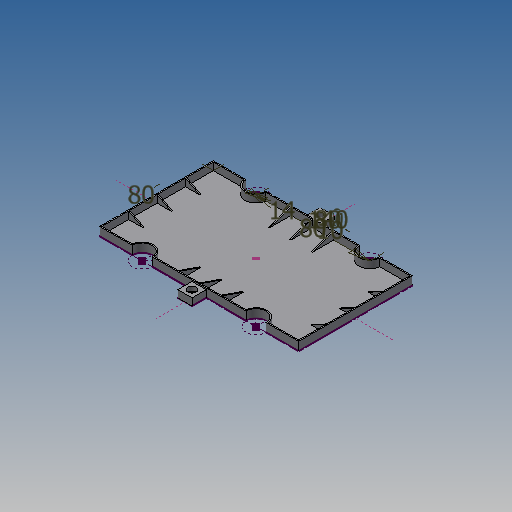
# Autodesk Inventor part: Leste_Meca_IIm_Ligne
Saved by Autodesk Inventor 2025.3 (Build 293356000, 356)
## iProperties
Created: 2026-08-27
Part Number: Leste_Meca_IIm_Ligne
Project: Nom Projet
Material: .
Description: Nom pièce
Document SubType Name: Modeling
Designer: jules
Authority: brut Ø
Mass: 0.0117645 g
Surface Area: 284.842 cm^2
Volume: 11.7645 cm^3
Density: 0.001 g/cm^3
Appearance: Par défaut
Material number: ---
Author: jules
Autodesk Inventor part; units mm, degrees
ref_plane "Plan YZ" through (0, 0, 0) normal (1, 0, 0) x (0, 1, 0)
ref_plane "Plan XZ" through (0, 0, 0) normal (0, 1, 0) x (-1, 0, 0)
ref_plane "Plan XY" through (0, 0, 0) normal (0, 0, 1) x (1, 0, 0)
sketch "Esquisse1" plane through (0, 0, 0) normal (0, 0, 1) x (1, 0, 0)
  line L0 (70, -40) -> (-70, -40) construction
  line L1 (-70, -40) -> (-70, 40)
  line L2 (-70, 40) -> (70, 40) construction
  line L3 (70, 40) -> (70, -40)
  line L4 (70, -40) -> (-70, 40) construction
  line L5 (-70, -40) -> (70, 40) construction
  line L6 (40, -40) -> (-40, -40) construction
  line L7 (-40, -40) -> (-40, 40) construction
  line L8 (-40, 40) -> (40, 40) construction
  line L9 (40, 40) -> (40, -40) construction
  line L10 (40, -40) -> (-40, 40) construction
  line L11 (-40, -40) -> (40, 40) construction
  circle A0 centre (-40, 40) radius 7 construction
  line L12 (-98, 0) -> (98, 0) construction
  arc A1 (-47, 40) -> (-33, 40) centre (-40, 40) ccw
  circle A2 centre (40, 40) radius 7 construction
  arc A3 (33, 40) -> (47, 40) centre (40, 40) ccw
  circle A4 centre (-40, -40) radius 7 construction
  arc A5 (-33, -40) -> (-47, -40) centre (-40, -40) ccw
  circle A6 centre (40, -40) radius 7 construction
  arc A7 (47, -40) -> (33, -40) centre (40, -40) ccw
  line L13 (-47, 40) -> (-70, 40)
  line L14 (-33, 40) -> (33, 40)
  line L15 (47, 40) -> (70, 40)
  line L16 (-70, -40) -> (70, -40) construction
  line L17 (-47, -40) -> (-70, -40)
  line L18 (-33, -40) -> (33, -40)
  line L19 (47, -40) -> (70, -40)
  line L20 (0, -70) -> (0, 70) construction
  line L21 (-5, 40) -> (5, 40)
  line L22 (5, 40) -> (5, 50)
  line L23 (5, 50) -> (-5, 50)
  line L24 (-5, 50) -> (-5, 40)
  line L25 (-5, 40) -> (5, 50) construction
  line L26 (5, 40) -> (-5, 50) construction
  line L27 (-70, -40) -> (70, -40) construction
  line L28 (-40, -40) -> (40, -40) construction
  line L29 (-33, -40) -> (33, -40)
  line L30 (5, -40) -> (5, -50)
  line L31 (5, -50) -> (-5, -50)
  line L32 (-5, -50) -> (-5, -40)
  point P0 (0, 0)
  point P1 (0, 45)
  dimension "d0" = 140
  dimension "d1" = 80
  dimension "d2" = 80
  dimension "d3" = 14
  dimension "d13" = 80
  dimension "d34" = 10
  dimension "d35" = 10
  constraints: 62 end point, 17 point on circle, 14 symmetric about line, 8 centre point, 6 midpoint, 6 parallel, 6 point on line, 4 collinear, 4 horizontal, 3 perpendicular, 1 coincident, 1 concentric, 1 vertical, 10 other
  measures "d0" distance of L1.end L2.end
  measures "d1" distance of L0.end L1.end
  measures "d2" distance of L7.end L8.end
  measures "d3" diameter of A0
  measures "d13" distance of A0.centre A2.centre
  measures "d34" distance of L23.end L22.end
  measures "d35" distance of L22.end L21.end
extrude "Extrusion1" add sketch "Esquisse1" along normal blind 6 contours L1 L13 A1 L14 A3 L15 L3 L19 A7 L18 A5 L17
shell "Coque1" thickness 0.8 removed faces 1 at (-11.5868, 11.786, 6)
sketch "Esquisse6" plane through (0, 0, 0) normal (1, 0, 0) x (0, 1, 0)
  line L0 (-39.2, 0.8) -> (-32.2, 0.8) construction
  line L1 (-39.2, 0.8) -> (-39.2, 6) construction
  line L2 (39.2, 0.8) -> (-39.2, 0.8) construction
  line L3 (-39.2, 0.8) -> (-39.2, 6) construction
  line L4 (-39.2, 6) -> (-24.2, 0.8)
  line L5 (-39.2, 0.8) -> (-39.2, 6)
  line L6 (-39.2, 0.8) -> (-24.2, 0.8)
  line L7 (0, -1.2) -> (0, 7.2) construction
  line L8 (39.2, 0.8) -> (32.2, 0.8) construction
  line L9 (39.2, 0.8) -> (39.2, 6) construction
  line L10 (-39.2, 0.8) -> (39.2, 0.8) construction
  line L11 (39.2, 0.8) -> (39.2, 6) construction
  line L12 (39.2, 6) -> (24.2, 0.8)
  line L13 (39.2, 0.8) -> (39.2, 6)
  line L14 (39.2, 0.8) -> (24.2, 0.8)
  point P0 (0, 0)
  dimension "d22" = 15
  constraints: 20 end point, 5 symmetric about line, 2 collinear, 2 point on line
  measures "d22" distance of L0.start L4.end
extrude "Extrusion2" add sketch "Esquisse6" along normal mid plane 0.8
pattern_linear "Réseau rectangulaire1" count 3 spacing 15 along (-1, 0, 0) of "Extrusion2" first direction both ways yes
sketch "Esquisse7" plane through (0, 0, 0) normal (0, 1, 0) x (-1, 0, 0)
  line L0 (69.2, 0.8) -> (69.2, 6) construction
  line L1 (47.7589, 0.8) -> (69.2, 0.8) construction
  line L2 (69.2, 6) -> (59.2, 0.8)
  line L3 (69.2, 0.8) -> (69.2, 6)
  line L4 (69.2, 0.8) -> (59.2, 0.8)
  line L5 (0, -1.2) -> (0, 7.2) construction
  line L6 (-69.2, 0.8) -> (-69.2, 6) construction
  line L7 (-47.7589, 0.8) -> (-69.2, 0.8) construction
  line L8 (-69.2, 6) -> (-59.2, 0.8)
  line L9 (-69.2, 0.8) -> (-69.2, 6)
  line L10 (-69.2, 0.8) -> (-59.2, 0.8)
  point P0 (0, 0)
  dimension "d28" = 10
  constraints: 16 end point, 4 symmetric about line, 2 point on line, 1 perpendicular, 1 vertical
  measures "d28" distance from line of L0 L2.end
extrude "Extrusion3" add sketch "Esquisse7" along normal mid plane 0.8
pattern_linear "Réseau rectangulaire2" count 3 spacing 20 along (0, -1, 0) of "Extrusion3" first direction both ways yes
extrude "Extrusion4" add sketch "Esquisse1" along normal blind 5 contours L18 L30 L31 L32 | L24 L23 L22 L14
sketch "Esquisse8" plane through (0, 0, 5) normal (0, 0, 1) x (1, 0, 0)
  line L0 (-5, 40) -> (5, 50) construction
  line L1 (5, 40) -> (-5, 50) construction
  point P0 (0, 0)
  point P1 (0, 45)
hole "Perçage1" at (0, 45, 5) direction (0, 0, -1) diameter 3.4 end through all start extended yes counterbore diameter 6 counterbore depth 3 clearance for "Vis d'assemblage à tête hexagonale ISO 24017" size "M3" standard "ISO"
mirror "Mise en miroir1" about plane through (0, 0, 0) normal (0, 1, 0) of "Perçage1"
